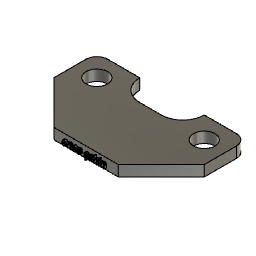
Model 18 (Autodesk Fusion 360 design; units mm, degrees)
Autodesk Fusion 360 part; units mm, degrees
sketch "Sketch1" plane through (0, 0, 0) normal (0, 0, 1) x (1, 0, 0)
  line L0 (20, 0) -> (50, 0)
  line L1 (70, 20) -> (70, 35)
  line L2 (35, 0) -> (20, 0) construction
  line L3 (0, 0) -> (0, 20) construction
  line L4 (35, 0) -> (50, 0) construction
  line L5 (20, 0) -> (0, 20)
  line L6 (50, 0) -> (70, 20)
  line L7 (0, 20) -> (0, 30) construction
  line L8 (70, 20) -> (70, 30) construction
  line L9 (0, 30) -> (10, 30) construction
  line L10 (70, 30) -> (60, 30) construction
  circle A0 centre (10, 30) radius 5
  arc A1 (5, 40) -> (0, 35) centre (5, 35) ccw
  arc A2 (70, 35) -> (65, 40) centre (65, 35) ccw
  line L11 (30, 30) -> (40, 30)
  arc A3 (20, 40) -> (30.003, 30) centre (30, 40) ccw
  arc A4 (40, 30) -> (50, 40) centre (40, 40) ccw
  line L12 (65, 40) -> (50, 40)
  line L13 (20, 40) -> (5, 40)
  line L14 (0, 0) -> (0, 20) construction
  line L15 (0, 0) -> (20, 0) construction
  line L16 (50, 0) -> (70, 0) construction
  line L17 (70, 0) -> (70, 20) construction
  line L18 (0, 35) -> (0, 30)
  line L19 (0, 30) -> (0, 20)
  circle A5 centre (60, 30) radius 5
  point P0 (0, 40)
  dimension "d1" = 70
  dimension "d2" = 40
  dimension "d3" = 15
  dimension "d4" = 20
  dimension "d5" = 15
  dimension "d6" = 20
  dimension "d9" = 30
  dimension "d10" = 30
  dimension "d11" = 10
  dimension "d12" = 10
  dimension "d13" = 10
  dimension "d14" = 5
  dimension "d15" = 5
  dimension "d18" = 20
  dimension "d20" = 10
  dimension "d21" = 10
  dimension "d22" = 20
  dimension "d23" = 30
  dimension "d24" = 10
  constraint horizontal L0
  constraint vertical L1
  constraint horizontal L12
  constraint vertical L18
  constraint coincident L3.start L14.start
  constraint parallel L0 L2
  constraint perpendicular L0 L3
  constraint parallel L2 L4
  constraint perpendicular L0 L7
  constraint perpendicular L0 L8
  constraint perpendicular L7 L9
  constraint perpendicular L8 L10
  constraint coincident L9.end A0.centre
  constraint coincident P0 L12
  constraint coincident P0 L18
  constraint tangent A1 L12
  constraint tangent A1 L18
  constraint tangent L1 A2
  constraint tangent A2 L12
  constraint tangent L11 A4
  constraint coincident L11 A3.end
  constraint coincident A3.start L12
  constraint collinear L12 L13
  constraint coincident L0 L2.start
  constraint parallel L2 L15
  constraint horizontal L16
  constraint vertical L17
  constraint coincident L10.end A5.centre
  measures "d1" distance of L3.start L16.end
  measures "d2" distance of L3.start P0
  measures "d3" distance of L2.start L0.start
  measures "d4" distance of L3.start L3.end
  measures "d5" distance of L2.start L0.end
  measures "d6" distance of L16.end L1.start
  measures "d9" distance of L3.start L7.end
  measures "d10" distance of L16.end L8.end
  measures "d11" distance of L7.end L9.end
  measures "d12" distance of L8.end L10.end
  measures "d13" diameter of A0
  measures "d14" radius of A1
  measures "d15" radius of A2
  measures "d18" diameter of A4
  measures "d20" distance of L11.start L11.end
  measures "d21" radius of A3
  measures "d22" distance of L3.start L0.start
  measures "d23" distance of A3.start A4.end
  measures "d24" diameter of A5
extrude "Extrude1" add sketch "Sketch1" along normal blind 5
ref_plane "WorkPlane1" through (35, 0, 2.5) normal (0, -1, 0) x (1, 0, 0)
sketch "Sketch2" plane through (35, 0, 2.5) normal (0, -1, 0) x (1, 0, 0)
  line L0 (-10.3504, -1.3909) -> (10.3505, -1.3898) construction
  line L1 (10.3505, -1.3898) -> (10.3504, 1.3909) construction
  line L2 (10.3504, 1.3909) -> (-10.3505, 1.3898) construction
  line L3 (-10.3505, 1.3898) -> (-10.3504, -1.3909) construction
  text T0 "enes şahin" font "Arial" height 3 align left top in box 20.7009 x 2.7807 at (-10.3504, -1.3909) x (1, 0.000049) y (-0.000049, 1) spacing 1
  constraint coincident origin
extrude "Extrude2" add sketch "Sketch2" along normal blind 1 text T0
